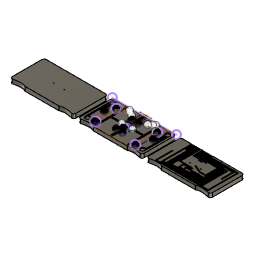
Arduino Foot Board V1.0 v3 (Autodesk Fusion 360 design; units mm, degrees)
Autodesk Fusion 360 part; units mm, degrees
(part 1 of 3)
sketch "TopZone" plane through (0, 0, 0) normal (0, 0, 1) x (1, 0, 0)
  line L0 (139.9424, 75.345) -> (-140.0576, 75.345)
  line L1 (-140.0576, 75.345) -> (-140.0576, -74.655)
  line L2 (-140.0576, -74.655) -> (139.9424, -74.655)
  line L3 (139.9424, -74.655) -> (139.9424, 75.345)
  line L4 (-0.0576, 75.345) -> (-0.0576, -74.655) construction
  line L5 (-140.0576, 0.345) -> (139.9424, 0.345) construction
  circle A0 centre (0, 0) radius 20
  circle A1 centre (0, 0) radius 27.5
  line L6 (-0.0576, 71.8935) -> (69.9424, 71.8935) construction
  line L7 (-0.0576, 71.8935) -> (-70.0576, 71.8935) construction
  line L8 (69.9424, 71.8935) -> (69.9424, -74.655)
  line L9 (69.9424, 71.8935) -> (69.9424, 75.345)
  line L10 (-70.0576, 71.8935) -> (-70.0576, 75.345)
  line L11 (-70.0576, 71.8935) -> (-70.0576, -74.655)
  line L12 (-8.6592, 0.345) -> (-8.6592, 2.845) construction
  line L13 (-8.6592, 0.345) -> (-8.6592, -2.155) construction
  line L14 (-27.3524, 2.845) -> (-70.0576, 2.845)
  line L15 (27.3524, 2.845) -> (69.9424, 2.845)
  line L16 (-27.4154, -2.155) -> (-70.0576, -2.155)
  line L17 (27.4154, -2.155) -> (69.9424, -2.155)
  line L18 (-0.0576, 7.4133) -> (2.4424, 7.4133) construction
  line L19 (-0.0576, 7.4133) -> (-5.0576, 7.4133) construction
  line L20 (4.9424, 27.0522) -> (4.9424, 75.345)
  line L21 (-5.0576, 27.0309) -> (-5.0576, 74.7158)
  line L22 (2.4424, -27.3913) -> (2.4424, -74.655)
  line L23 (-2.4424, -27.3913) -> (-2.4424, -74.655)
  line L24 (-0.0576, 48.2777) -> (4.9424, 48.2777) construction
  line L25 (-0.0576, 48.2777) -> (-5.0576, 48.2777) construction
  line L26 (41.5082, 0.345) -> (41.5082, 2.845) construction
  line L27 (41.5082, 0.345) -> (41.5082, -2.155) construction
  line L28 (-2.4424, -51.0232) -> (-0.0576, -51.0232) construction
  line L29 (-0.0576, -51.0232) -> (2.4424, -51.0232) construction
  line L30 (-47.1449, 0.345) -> (-47.1449, 2.845) construction
  line L31 (-47.1449, 0.345) -> (-47.1449, -2.155) construction
  line L32 (-0.0576, 41.5581) -> (85.9424, 41.5581) construction
  line L33 (-0.0576, 41.5581) -> (-86.0576, 41.5581) construction
  line L34 (-78.5277, 75.345) -> (-78.5277, 41.345) construction
  line L35 (-0.0576, -53.0508) -> (85.9424, -53.0508) construction
  line L36 (-86.0576, -53.0508) -> (-0.0576, -53.0508) construction
  line L37 (-80.4186, -74.655) -> (-80.4186, -54.655) construction
  line L38 (74.9056, 7.4117) -> (139.9424, 7.4117) construction
  line L39 (-75.019, 7.4166) -> (-140.0576, 7.4166) construction
  circle A2 centre (107.424, 7.4117) radius 12.5
  circle A3 centre (-107.5383, 7.4166) radius 12.5
  line L40 (-120.0383, 7.4166) -> (-120.0383, 57.4402) construction
  line L41 (-120.0383, 7.4166) -> (-120.0383, -52.5834) construction
  circle A4 centre (-120.0383, 57.4402) radius 10
  circle A5 centre (-120.0383, -52.5834) radius 10
  line L42 (-130.0383, -52.5834) -> (-130.0383, -52.5836)
  line L43 (-130.0383, 57.4402) -> (-130.0383, -52.5834)
  line L44 (-120.0383, 7.4166) -> (-120.0383, 47.4402)
  line L45 (-115.0383, 17.4167) -> (-115.0383, 47.4132)
  line L46 (-125.0305, 48.7754) -> (-125.0305, -43.9186)
  line L47 (-134.9926, -52.9708) -> (-134.9926, -52.2027)
  line L48 (-115.0383, 47.4132) -> (-115.0383, 48.7799)
  line L49 (119.924, 7.4117) -> (119.924, 57.4123) construction
  line L50 (119.924, 7.4117) -> (119.924, -52.5883) construction
  circle A6 centre (119.924, 57.4112) radius 10
  circle A7 centre (119.924, -52.5883) radius 10
  line L51 (129.924, -52.5895) -> (129.924, 57.4112)
  line L52 (119.924, 7.4117) -> (119.924, 47.4112)
  line L53 (114.9249, 17.411) -> (114.9249, 47.4133)
  line L54 (124.9251, -43.9287) -> (124.9251, 48.7516)
  line L55 (114.9249, 47.4133) -> (114.9249, 48.7504)
  line L56 (2.4424, -74.655) -> (13.049, -64.0484) construction
  line L57 (2.4424, -74.655) -> (17.5, -74.655) construction
  line L58 (-2.4424, -74.655) -> (-13.049, -64.0484) construction
  line L59 (-2.4424, -74.655) -> (12.5, -74.655) construction
  line L60 (4.9424, 75.345) -> (15.549, 64.7384) construction
  line L61 (4.9424, 75.345) -> (17.5, 75.345) construction
  line L62 (-5.0576, 74.7158) -> (-15.6642, 64.1092) construction
  line L63 (-5.0576, 74.7158) -> (12.5, 74.7158) construction
  circle A8 centre (13.049, -34.0489) radius 1.55
  circle A9 centre (-13.049, -34.0489) radius 1.55
  circle A10 centre (13.049, 34.7379) radius 1.55
  circle A11 centre (-13.1642, 34.387) radius 1.55
  circle A12 centre (-107.5383, 7.4166) radius 1.55
  circle A13 centre (107.424, 7.4117) radius 1.55
  circle A14 centre (0, 0) radius 1.55
  circle A15 centre (0, 0) radius 4
  circle A16 centre (13.049, -34.0489) radius 4
  circle A17 centre (-13.049, -34.0489) radius 4
  circle A18 centre (13.049, 34.7379) radius 4
  circle A19 centre (-13.1642, 34.387) radius 4
  circle A20 centre (107.424, 7.4117) radius 4
  circle A21 centre (-107.5383, 7.4166) radius 4
  line L64 (-75.019, 71.8935) -> (-75.019, -74.6555)
  line L65 (74.9056, 71.8935) -> (74.9056, -74.6555)
  line L66 (74.9056, 71.8935) -> (74.9056, 75.345)
  line L67 (-75.019, 71.8935) -> (-75.019, 75.345)
  line L68 (-5.0576, 74.7158) -> (-5.0576, 75.345)
  line L69 (74.9056, 7.4117) -> (-75.019, 7.4166) construction
  line L70 (-13.1642, 64.387) -> (-13.1642, 44.387) construction
  line L71 (13.049, 64.7379) -> (13.049, 44.7379) construction
  line L72 (-13.049, -64.0489) -> (-13.049, -44.0489) construction
  line L73 (13.049, -64.0489) -> (13.049, -44.0489) construction
  point P0 (-0.0576, -74.655)
  point P1 (-0.0576, 75.345)
  point P2 (139.9424, 0.345)
  point P3 (-140.0576, 0.345)
  dimension "d1" = 280
  dimension "d2" = 150
  dimension "d3" = 40
  dimension "d4" = 55
  dimension "d5" = 70
  dimension "d6" = 70
  dimension "d9" = 2.5
  dimension "d10" = 2.5
  dimension "d11" = 5
  dimension "d12" = 5
  dimension "d13" = 5
  dimension "d14" = 2.5
  dimension "d15" = 2.5
  dimension "d16" = 2.5
  dimension "d18" = 2.5
  dimension "d19" = 2.5
  dimension "d20" = 86
  dimension "d24" = 34
  dimension "d25" = 20
  dimension "d26" = 25
  dimension "d27" = 25
  dimension "d29" = 60
  dimension "d30" = 20
  dimension "d31" = 20
  dimension "d35" = 60
  dimension "d36" = 20
  dimension "d37" = 20
  dimension "d40" = 15
  dimension "d41" = 45
  dimension "d42" = 135
  dimension "d43" = 15
  dimension "d44" = 15
  dimension "d45" = 45
  dimension "d46" = 135
  dimension "d47" = 15
  dimension "d50" = 3.1
  dimension "d51" = 3.1
  dimension "d52" = 3.1
  dimension "d53" = 3.1
  dimension "d54" = 3.1
  dimension "d55" = 3.1
  dimension "d56" = 3.1
  dimension "d58" = 8
  dimension "d59" = 8
  dimension "d60" = 8
  dimension "d61" = 8
  dimension "d62" = 8
  dimension "d63" = 8
  dimension "d64" = 8
  dimension "d133" = 20
  dimension "d134" = 20
  dimension "d135" = 20
  dimension "d136" = 20
  constraint horizontal L0
  constraint perpendicular L0 L1
  constraint parallel L0 L2
  constraint parallel L1 L3
  constraint coincident A0.centre A1.centre
  constraint midpoint L0 P1
  constraint midpoint L2 P0
  constraint midpoint L1 P3
  constraint midpoint L3 P2
  constraint coincident L4 L6.start
  constraint perpendicular L4 L6
  constraint perpendicular L4 L7
  constraint coincident L2 L8.end
  constraint perpendicular L2 L8
  constraint coincident L0 L9.end
  constraint perpendicular L0 L9
  constraint coincident L0 L10.end
  constraint perpendicular L0 L10
  constraint coincident L2 L11.end
  constraint perpendicular L2 L11
  constraint coincident L5 L12.start
  constraint perpendicular L5 L12
  constraint perpendicular L5 L13
  constraint equal L12 L13
  constraint coincident A1 L14.start
  constraint coincident L11 L14.end
  constraint perpendicular L11 L14
  constraint coincident A1 L15.start
  constraint coincident L8 L15.end
  constraint perpendicular L8 L15
  constraint coincident A1 L16.start
  constraint coincident L11 L16.end
  constraint perpendicular L11 L16
  constraint coincident A1 L17.start
  constraint coincident L8 L17.end
  constraint perpendicular L8 L17
  constraint coincident L4 L18.start
  constraint perpendicular L4 L18
  constraint perpendicular L4 L19
  constraint coincident A1 L20.start
  constraint coincident L0 L20.end
  constraint perpendicular L0 L20
  constraint coincident A1 L21.start
  constraint perpendicular L19 L21
  constraint coincident A1 L22.start
  constraint coincident L2 L22.end
  constraint perpendicular L2 L22
  constraint coincident A1 L23.start
  constraint coincident L2 L23.end
  constraint perpendicular L2 L23
  constraint coincident L4 L24.start
  constraint coincident L20 L24.end
  constraint perpendicular L20 L24
  constraint coincident L21 L25.end
  constraint perpendicular L21 L25
  constraint coincident P0 L4.end
  constraint coincident P1 L4.start
  constraint coincident P2 L5.end
  constraint coincident P3 L5.start
  constraint coincident L5 L26.start
  constraint coincident L15 L26.end
  constraint perpendicular L15 L26
  constraint coincident L17 L27.end
  constraint perpendicular L17 L27
  constraint midpoint L23 L28.start
  constraint coincident L4 L28.end
  constraint perpendicular L23 L28
  constraint midpoint L22 L29.end
  constraint perpendicular L22 L29
  constraint coincident L5 L30.start
  constraint coincident L14 L30.end
  constraint perpendicular L14 L30
  constraint coincident L16 L31.end
  constraint perpendicular L16 L31
  constraint coincident L4 L32.start
  constraint perpendicular L32 L65
  constraint perpendicular L33 L64
  constraint coincident L0 L34.start
  constraint perpendicular L0 L34
  constraint coincident L4 L35.start
  constraint perpendicular L35 L65
  constraint perpendicular L4 L36
  constraint equal L32 L33
  constraint equal L32 L35
  constraint equal L32 L36
  constraint coincident L2 L37.start
  constraint perpendicular L36 L37
  constraint coincident L38.start L65
  constraint coincident L3 L38.end
  constraint perpendicular L3 L38
  constraint coincident L39.start L64
  constraint coincident L1 L39.end
  constraint perpendicular L1 L39
  constraint midpoint L38 A2.centre
  constraint midpoint L39 A3.centre
  constraint coincident A3 L40.start
  constraint coincident L39 L40.start
  constraint perpendicular L39 L40
  constraint perpendicular L5 L41
  constraint coincident L40.end A4.centre
  constraint coincident L41.end A5.centre
  constraint coincident A5 L42.start
  constraint coincident A5 L42.end
  constraint vertical L42
  constraint coincident A4 L43.start
  constraint perpendicular L5 L43
  constraint coincident A4 L44.end
  constraint coincident L40 L44.end
  constraint parallel L43 L46
  constraint parallel L42 L47
  constraint coincident A4 L46.start
  constraint coincident A5 L46.end
  constraint parallel L44 L45
  constraint coincident A3 L45.start
  constraint coincident A4 L48.end
  constraint parallel L45 L48
  constraint tangent A4 L43
  constraint tangent A5 L43
  constraint coincident A2 L49.start
  constraint coincident L38 L49.start
  constraint perpendicular L38 L49
  constraint perpendicular L38 L50
  constraint coincident L50.end A7.centre
  constraint coincident A7 L51.start
  constraint coincident A6 L51.end
  constraint tangent A6 L51
  constraint coincident A6 L52.end
  constraint perpendicular L38 L52
  constraint coincident A6 L55.end
  constraint parallel L53 L55
  constraint parallel L51 L54
  constraint coincident A6 L54.end
  constraint parallel L52 L53
  constraint coincident A2 L53.start
  constraint coincident A7 L54.start
  constraint horizontal L57
  constraint horizontal L59
  constraint horizontal L61
  constraint horizontal L63
  constraint concentric A3 A12
  constraint concentric A2 A13
  constraint concentric A1 A14
  constraint concentric A0 A15
  constraint concentric A8 A16
  constraint concentric A9 A17
  constraint concentric A10 A18
  constraint concentric A11 A19
  constraint concentric A13 A20
  constraint concentric A3 A21
  constraint parallel L8 L65
  constraint parallel L11 L64
  constraint coincident L0 L66.end
  constraint perpendicular L0 L66
  constraint coincident L0 L67.end
  constraint perpendicular L0 L67
  constraint coincident L0 L68.end
  constraint perpendicular L0 L68
  constraint vertical L70
  constraint vertical L71
  constraint perpendicular L36 L72
  constraint vertical L73
  measures "d1" distance of L1.end L2.end
  measures "d2" distance of L0.end L1.end
  measures "d3" diameter of A0
  measures "d4" diameter of A1
  measures "d5" distance of L6.start L6.end
  measures "d6" distance of L6.start L7.end
  measures "d9" distance of L12.start L12.end
  measures "d10" distance of L18.start L18.end
  measures "d11" distance of L18.start L19.end
  measures "d12" distance of L24.start L24.end
  measures "d13" distance of L24.start L25.end
  measures "d14" distance of L26.start L26.end
  measures "d15" distance of L26.start L27.end
  measures "d16" distance of L30.start L30.end
  measures "d18" distance of L30.start L31.end
  measures "d19" distance of L28.end L29.end
  measures "d20" distance of L32.start L32.end
  measures "d24" distance of L34.start L34.end
  measures "d25" distance of L37.start L37.end
  measures "d26" diameter of A2
  measures "d27" diameter of A3
  measures "d29" distance of L40.start L41.end
  measures "d30" diameter of A4
  measures "d31" diameter of A5
  measures "d35" distance of L49.start L50.end
  measures "d36" diameter of A6
  measures "d37" diameter of A7
  measures "d40" distance of L22.end L56.end
  measures "d41" angle of L56 L57
  measures "d42" angle of L58 L59
  measures "d43" distance of L23.end L58.end
  measures "d44" distance of L20.end L60.end
  measures "d45" angle of L60 L61
  measures "d46" angle of L62 L63
  measures "d47" distance of L21.end L62.end
  measures "d50" diameter of A8
  measures "d51" diameter of A9
  measures "d52" diameter of A10
  measures "d53" diameter of A11
  measures "d54" diameter of A12
  measures "d55" diameter of A13
  measures "d56" diameter of A14
  measures "d58" diameter of A15
  measures "d59" diameter of A16
  measures "d60" diameter of A17
  measures "d61" diameter of A18
  measures "d62" diameter of A19
  measures "d63" diameter of A20
  measures "d64" diameter of A21
  measures "d133" distance of L70.start L70.end
  measures "d134" distance of L71.start L71.end
  measures "d135" distance of L72.start L72.end
  measures "d136" distance of L73.start L73.end
sketch "LightResistorMeasurement" plane through (0, 0, 0) normal (0, 0, 1) x (1, 0, 0) in component "LightResistor v3"
  line L0 (0, 0) -> (0.0874, 0)
  line L1 (0, 0) -> (0, 2) construction
  line L2 (0, 0) -> (0, -2) construction
  line L3 (0, 2) -> (1.5, 2)
  line L4 (0, 2) -> (-1.5, 2)
  line L5 (0, -2) -> (1.5, -2)
  line L6 (0, -2) -> (-1.5, -2)
  arc A0 (-1.5, 2) -> (-1.5, -2) centre (0, 0) ccw
  arc A1 (1.5, -2) -> (1.5, 2) centre (0, 0) ccw
  line L7 (0, 0) -> (2, 0) construction
  line L8 (0, 0) -> (-2, 0) construction
  circle A2 centre (-1.7, 0) radius 0.3
  circle A3 centre (1.7, 0) radius 0.3
  dimension "d1_1" = 5
  dimension "d2_1" = 2
  dimension "d3_1" = 2
  dimension "d4_1" = 2
  dimension "d5_1" = 0.6
  dimension "d6_1" = 0.6
  constraint coincident L0.start L1.start
  constraint horizontal L0
  constraint perpendicular L0 L1
  constraint perpendicular L0 L2
  constraint equal L1 L2
  constraint perpendicular L1 L3
  constraint perpendicular L1 L4
  constraint coincident L5.end A0
  constraint perpendicular L2 L5
  constraint perpendicular L2 L6
  constraint concentric A0 A1
  constraint perpendicular L1 L7
  constraint perpendicular L2 L8
  constraint coincident L8.end A2
  constraint coincident L7.end A3
  measures "d1_1" diameter of A0
  measures "d2_1" distance of L0.start L1.end
  measures "d3_1" distance of L0.start L7.end
  measures "d4_1" distance of L0.start L8.end
  measures "d5_1" diameter of A2
  measures "d6_1" diameter of A3
extrude "Extrude1" add sketch "LightResistorMeasurement" along normal blind 1.8 contours L3 L4 L5 L6 A0 A1 | A2 | A3 makes body 1 in component "LightResistor v3"
extrude "Extrude2" add sketch "LightResistorMeasurement" against normal blind 24 contours A2 | A3 bodies 1 in component "LightResistor v3"
extrude "Extrude3" add sketch "LightResistorMeasurement" along normal blind 2 contours A2 | A3 bodies 1 in component "LightResistor v3"
sketch "WoodBoard" plane through (0, 0, 0) normal (0, 0, 1) x (1, 0, 0)
  line L0 (140, 75) -> (-140, 75)
  line L1 (-140, 75) -> (-140, -75)
  line L2 (-140, -75) -> (140, -75)
  line L3 (140, -75) -> (140, 75)
  line L4 (140, 75) -> (-140, -75) construction
  line L5 (-140, 75) -> (140, -75) construction
  dimension "d65" = 280
  dimension "d66" = 150
  constraint horizontal L0
  constraint perpendicular L0 L1
  constraint parallel L0 L2
  constraint parallel L1 L3
  constraint coincident L4 origin
  constraint coincident L5 origin
  measures "d65" distance of L1.end L2.end
  measures "d66" distance of L0.end L1.end
extrude "Extrude1'" add sketch "WoodBoard" against normal blind 18 separate body makes body 2
copy_body "CutPasteBodies1" bodies 1 removing the originals makes body 3
copy_body "CopyPasteBodies2" bodies 3 makes body 4
move_body "Move1" bodies 4 to x (1, 0, 0) y (0, 1, 0) z (0, 0, 1) at (-86.0576, 41.5581, 0)
copy_body "CopyPasteBodies3" bodies 3 makes body 5
move_body "Move2" bodies 5 to x (1, 0, 0) y (0, 1, 0) z (0, 0, 1) at (85.9424, 41.5581, 0)
copy_body "CopyPasteBodies4" bodies 3 makes body 6
move_body "Move3" bodies 6 to x (1, 0, 0) y (0, 1, 0) z (0, 0, 1) at (-86.0576, -53.0508, 0)
copy_body "CopyPasteBodies5" bodies 3 makes body 7
move_body "Move4" bodies 7 to x (1, 0, 0) y (0, 1, 0) z (0, 0, 1) at (85.9424, -53.0508, 0)
move_body "Move5" bodies 3 6 5 4 7 to x (1, 0, 0) y (0, 1, 0) z (0, 0, 1) at (0, 0, -1.8)
move_body "Move6" bodies 3 to x (1, 0, 0) y (0, 1, 0) z (0, 0, 1) at (0, -17, 0)
combine "Combine1" operation cut target body 2 tool bodies 3 4 5 6 7
sketch "LightResistorHoles" plane through (0, 0, 0) normal (0, 0, 1) x (1, 0, 0)
  circle A0 centre (-86.0576, 41.5581) radius 3
  circle A1 centre (85.9424, 41.5581) radius 3
  circle A2 centre (85.9424, -53.0508) radius 3
  circle A3 centre (-86.0576, -53.0508) radius 3
  circle A4 centre (-84.3576, 41.5581) radius 0.3
  circle A5 centre (-89.3076, 41.5581) radius 1.55
  circle A6 centre (-87.7576, 41.5581) radius 0.3
  circle A7 centre (-82.8076, -53.0508) radius 1.55
  circle A8 centre (-84.3576, -53.0508) radius 0.3
  circle A9 centre (-89.3065, -53.1098) radius 1.55
  circle A10 centre (-87.7576, -53.0508) radius 0.3
  circle A11 centre (89.1924, -53.0508) radius 1.55
  circle A12 centre (87.6424, -53.0508) radius 0.3
  circle A13 centre (82.6924, -53.0508) radius 1.55
  circle A14 centre (84.2424, -53.0508) radius 0.3
  circle A15 centre (89.1924, 41.5581) radius 1.55
  circle A16 centre (87.6424, 41.5581) radius 0.3
  circle A17 centre (82.6924, 41.5581) radius 1.55
  circle A18 centre (84.2424, 41.5581) radius 0.3
  circle A19 centre (2.6428, -15.7697) radius 1.55
  circle A20 centre (1.7, -17) radius 0.3
  circle A21 centre (-2.655, -15.7792) radius 1.55
  circle A22 centre (-1.7, -17) radius 0.3
  circle A23 centre (-82.8076, 41.5581) radius 1.55
  line L0 (-1.5, -15) -> (1.5, -15)
  line L1 (0, -15) -> (0, -13) construction
  circle A24 centre (0, 0) radius 20
  line L2 (0, -13) -> (15.1987, -13)
  line L3 (0, -13) -> (-15.1987, -13)
  line L4 (0, -13) -> (0, -11) construction
  line L5 (0, -11) -> (16.7033, -11)
  line L6 (0, -11) -> (-16.7033, -11)
  circle A25 centre (-86.0576, 41.5581) radius 4.8
  circle A26 centre (-86.0576, 41.5581) radius 6.5
  circle A27 centre (-86.0576, -53.0508) radius 4.8
  circle A28 centre (-86.0576, -53.0508) radius 6.5
  circle A29 centre (85.9424, -53.0508) radius 4.7714
  circle A30 centre (85.9424, -53.0508) radius 6.5
  circle A31 centre (85.9424, 41.5581) radius 4.8
  circle A32 centre (85.9424, 41.5581) radius 6.5
  point P0 (-86.0576, 41.5581)
  point P1 (85.9424, 41.5581)
  point P2 (85.9424, -53.0508)
  point P3 (-86.0576, -53.0508)
  dimension "d70" = 6
  dimension "d75" = 3.1
  dimension "d76" = 3.1
  dimension "d77" = 3.1
  dimension "d78" = 3.1
  dimension "d79" = 3.1
  dimension "d80" = 3.1
  dimension "d81" = 3.1
  dimension "d82" = 3.1
  dimension "d83" = 3.1
  dimension "d84" = 3.1
  dimension "d97" = 2
  dimension "d98" = 2
  dimension "d101" = 13
  constraint coincident P0 A0.centre
  constraint coincident P1 A1.centre
  constraint coincident P2 A2.centre
  constraint coincident P3 A3.centre
  constraint equal A0 A1
  constraint equal A0 A3
  constraint equal A0 A2
  constraint coincident A5 A6.centre
  constraint coincident A7 A8.centre
  constraint coincident A9 A10.centre
  constraint coincident A11 A12.centre
  constraint coincident A13 A14.centre
  constraint coincident A15 A16.centre
  constraint coincident A17 A18.centre
  constraint coincident A19 A20.centre
  constraint coincident A21 A22.centre
  constraint coincident A4.centre A23
  constraint midpoint L0 L1.start
  constraint perpendicular L0 L1
  constraint coincident A24 L2.end
  constraint perpendicular L1 L2
  constraint coincident A24 L3.end
  constraint perpendicular L1 L3
  constraint perpendicular L3 L4
  constraint coincident A24 L5.end
  constraint perpendicular L4 L5
  constraint coincident A24 L6.end
  constraint perpendicular L4 L6
  constraint tangent A23 A25
  constraint concentric A25 A26
  constraint concentric A3 A27
  constraint tangent A7 A27
  constraint concentric A2 A29
  constraint concentric A29 A30
  constraint concentric A1 A31
  constraint tangent A15 A31
  constraint concentric A1 A32
  constraint equal A26 A28
  constraint equal A26 A30
  constraint equal A26 A32
  measures "d70" diameter of A0
  measures "d75" diameter of A5
  measures "d76" diameter of A7
  measures "d77" diameter of A9
  measures "d78" diameter of A11
  measures "d79" diameter of A13
  measures "d80" diameter of A15
  measures "d81" diameter of A17
  measures "d82" diameter of A19
  measures "d83" diameter of A21
  measures "d84" diameter of A23
  measures "d97" distance of L1.start L1.end
  measures "d98" distance of L1.end L4.end
  measures "d101" diameter of A26
extrude "Extrude2'" cut sketch "LightResistorHoles" against normal blind 18 contours A0 A4 A23 | A0 A23 | A0 A5 A6 | A0 A5 | A4 A23 | A5 A6 | A1 A15 A16 | A1 A15 | A1 A17 A18 | A1 A17 | A15 A16 | A17 A18 | A2 A11 A12 | A2 A11 A29 | A2 A13 A14 | A2 A13 A29 | A11 A29 | A11 A12 | A13 A14 | A13 A29 | A3 A7 A8 | A3 A7 | A3 A9 A10 | A3 A9 | A7 A8 | A9 A10 | A19 A20 | A19 A20 | A21 A22 | A21 A22 picked at (-84.2555, 41.5581) picked at (-87.8544, 41.6205) picked at (87.7445, 41.5581) picked at (84.1456, 41.4957) picked at (87.7445, -53.0508) picked at (84.1456, -52.9883) picked at (-84.2555, -53.0508) picked at (-87.8583, -53.054) picked at (2.9931, -15.2653) picked at (1.7637, -16.9202) picked at (-3.0046, -15.274) picked at (-1.7629, -16.9195) bodies 2
extrude "Extrude3'" cut sketch "TopZone" against normal blind 1 contours L0 L2 L3 L65 L66 | L0 A1 L8 L9 L15 L20 | L2 A1 L8 L17 L22 | L0 A1 L10 L11 L14 L21 L68 | L2 A1 L11 L16 L23 | L0 L1 L2 L64 L67 | A0 bodies 2
extrude "Extrude4" cut sketch "TopZone" against normal blind 2 contours A15 | A16 | A17 | A18 | A19 | A20 | A21 bodies 2
extrude "Extrude5" cut sketch "TopZone" against normal blind 18 contours A8 | A9 | A10 | A11 | A12 | A13 | A14 bodies 2
extrude "Extrude6" cut sketch "TopZone" against normal blind 5 contours A2 | A2 A6 L52 L53 L55 | A6 | A6 A7 L51 L54 | A7 | A3 | A3 A4 L44 L45 L48 | A4 | A4 A5 L43 L46 | A5 bodies 2
extrude "Extrude7" cut sketch "TopZone" against normal blind 6 contours A20 | A21 bodies 2
extrude "Extrude8" add sketch "LightResistorHoles" against normal blind 3 contours A24 L2 L3 L5 L6 bodies 2
extrude "Extrude9" add sketch "LightResistorHoles" against normal blind 2 contours A26 | A28 | A30 | A32 bodies 2
sketch "RefPoints" plane through (0, 0, 0) normal (0, 0, 1) x (1, 0, 0)
  line L0 (-140, 75) -> (140, 75)
  line L1 (0, 0) -> (0, 81.0594) construction
  circle A0 centre (13.049, 34.7379) radius 1.55 construction
  line L2 (13.049, 34.7379) -> (13.049, 81.0594) construction
  circle A1 centre (-13.1642, 34.387) radius 1.55 construction
  line L3 (-13.1642, 34.387) -> (-13.1642, 81.0594) construction
  line L4 (0, 81.0594) -> (13.049, 81.0594) construction
  line L5 (0, 81.0594) -> (-13.1642, 81.0594) construction
  line L6 (6.5245, 81.0594) -> (6.5245, -71.9033) construction
  line L7 (6.5245, -71.9033) -> (78.613, -71.9033) construction
  line L8 (6.5245, -71.9033) -> (-78.7073, -71.9033) construction
  line L9 (82.8285, 41.5581) -> (82.8285, -53.0508) construction
  line L10 (82.8285, -53.0508) -> (82.8285, -71.9033) construction
  line L11 (78.613, -71.9033) -> (82.8285, -71.9033) construction
  arc A2 (-84.3286, -53.3494) -> (-84.3286, -52.7522) centre (-82.8076, -53.0508) ccw construction
  line L12 (-82.8598, 41.5581) -> (-82.8076, -53.0508) construction
  line L13 (-82.8076, -53.0508) -> (-82.7972, -71.9033) construction
  line L14 (-82.7972, -71.9033) -> (-78.7073, -71.9033) construction
  arc A3 (-88.2745, 42.7136) -> (-90.8576, 41.5581) centre (-89.3076, 41.5581) ccw construction
  line L15 (-89.3076, 41.5581) -> (-89.3076, 50.5559) construction
  arc A4 (90.7424, 41.5581) -> (88.1593, 42.7136) centre (89.1924, 41.5581) ccw construction
  line L16 (89.1924, 41.5581) -> (89.1924, 50.5559) construction
  arc A5 (88.1593, -54.2063) -> (90.7002, -53.4097) centre (89.1924, -53.0508) ccw construction
  line L17 (89.1924, -53.0508) -> (99.1924, -53.0508) construction
  arc A6 (-87.798, -52.7535) -> (-87.7753, -53.3502) centre (-89.3065, -53.1098) ccw construction
  line L18 (-89.3065, -53.1098) -> (-99.306, -53.2065) construction
  line L19 (-99.306, -53.2065) -> (-100.3741, 57.1678) construction
  circle A7 centre (-107.5383, 7.4166) radius 1.55 construction
  line L20 (-107.5383, 7.4166) -> (-107.5383, 65.4886) construction
  line L21 (99.1924, -53.0508) -> (99.1924, 59.674) construction
  circle A8 centre (107.424, 7.4117) radius 1.55 construction
  line L22 (107.424, 7.4117) -> (107.424, 65.1009) construction
  line L23 (107.424, 65.1009) -> (59.9835, 65.1009) construction
  line L24 (99.1924, 59.674) -> (50.873, 59.674) construction
  line L25 (89.1924, 50.5559) -> (38.3153, 50.5559) construction
  line L26 (-89.3076, 50.5559) -> (-31.1213, 50.5559) construction
  arc A9 (1.9547, -17.1586) -> (1.4807, -16.7953) centre (2.6428, -15.7697) ccw construction
  line L27 (2.6428, -15.7697) -> (6.5245, -15.7697) construction
  arc A10 (-1.4827, -16.7932) -> (-1.9531, -17.1611) centre (-2.655, -15.7792) ccw construction
  line L28 (-2.655, -15.7792) -> (-6.5367, -15.7792) construction
  line L29 (-6.5367, -15.7792) -> (-6.5367, 75.0019) construction
  line L30 (-6.5367, 75.0019) -> (-6.5821, 81.0594) construction
  line L31 (-100.3741, 57.1678) -> (-45.5643, 57.6981) construction
  line L32 (-107.5383, 65.4886) -> (-54.9128, 65.4886) construction
  circle A11 centre (-23.3525, 0) radius 1.55
  circle A12 centre (23.3525, 0) radius 1.55
  circle A13 centre (-13.049, -34.0489) radius 1.55
  line L33 (-13.049, -34.0489) -> (-23.049, -34.0489) construction
  circle A14 centre (13.049, -34.0489) radius 1.55
  line L34 (13.049, -34.0489) -> (23.049, -34.0489) construction
  line L35 (-23.049, -34.0489) -> (-23.049, 81.0594) construction
  line L36 (-23.049, 81.0594) -> (-13.1642, 81.0594) construction
  line L37 (23.049, -34.0489) -> (23.049, 81.0594) construction
  line L38 (23.049, 81.0594) -> (13.049, 81.0594) construction
  dimension "d107" = 10
  dimension "d108" = 10
  dimension "d109" = 3.1
  dimension "d110" = 3.1
  dimension "d131" = 10
  dimension "d132" = 10
  constraint coincident L1.start origin
  constraint perpendicular L0 L1
  constraint coincident A0.centre L2.start
  constraint perpendicular L0 L2
  constraint coincident A1.centre L3.start
  constraint perpendicular L0 L3
  constraint perpendicular L2 L4
  constraint perpendicular L3 L5
  constraint midpoint L4 L6.start
  constraint perpendicular L0 L6
  constraint perpendicular L6 L7
  constraint perpendicular L6 L8
  constraint perpendicular L8 L9
  constraint perpendicular L8 L10
  constraint perpendicular L10 L11
  constraint coincident A2.centre L12.end
  constraint parallel L8 L14
  constraint coincident A3.centre L15.start
  constraint perpendicular L8 L15
  constraint coincident A4.centre L16.start
  constraint coincident A5.centre L17.start
  constraint horizontal L17
  constraint coincident A6.centre L18.start
  constraint perpendicular L18 L19
  constraint vertical L20
  constraint coincident A7.centre L20.start
  constraint vertical L21
  constraint coincident A8.centre L22.start
  constraint perpendicular L17 L22
  constraint perpendicular L22 L23
  constraint perpendicular L21 L24
  constraint perpendicular L16 L25
  constraint perpendicular L15 L26
  constraint coincident A9.centre L27.start
  constraint coincident L6 L27.end
  constraint perpendicular L6 L27
  constraint coincident A10.centre L28.start
  constraint parallel L27 L28
  constraint equal L27 L28
  constraint vertical L29
  constraint midpoint L5 L30.end
  constraint perpendicular L19 L31
  constraint perpendicular L20 L32
  constraint coincident A13.centre L33.start
  constraint horizontal L33
  constraint coincident A14.centre L34.start
  constraint horizontal L34
  constraint perpendicular L5 L35
  constraint perpendicular L1 L36
  constraint perpendicular L0 L37
  constraint perpendicular L2 L38
  measures "d107" distance of A5.centre L17.end
  measures "d108" distance of A6.centre L18.end
  measures "d109" diameter of A11
  measures "d110" diameter of A12
  measures "d131" distance of A13.centre L33.end
  measures "d132" distance of A14.centre L34.end
extrude "Extrude10" cut sketch "RefPoints" against normal blind 2 contours A11 | A12 bodies 2
sketch "CutAround" plane through (0, 0, 0) normal (0, 0, 1) x (1, 0, 0)
  line L0 (-73.8561, -74.9863) -> (73.7471, -74.9863)
  line L1 (140, -64.9863) -> (140, 65)
  line L2 (130, 75) -> (-130, 75)
  line L3 (-140, 65) -> (-140, -64.9863)
  arc A0 (-130, 75) -> (-140, 65) centre (-130, 65) ccw
  arc A1 (140, 65) -> (130, 75) centre (130, 65) ccw
  arc A2 (-140, -64.9863) -> (-130.0009, -74.9863) centre (-130, -64.9863) ccw
  arc A3 (130.0008, -74.9863) -> (140, -64.9863) centre (130, -64.9863) ccw
  line L4 (-75.019, -74.655) -> (-140, -74.655)
  line L5 (-107.5095, -74.655) -> (-107.5095, -70.655) construction
  line L6 (139.9424, -74.655) -> (74.9056, -74.655)
  line L7 (107.424, -74.655) -> (107.424, -70.655) construction
  spline S0 degree 5 poles (-130.0009, -74.9863) (-129.11, -74.7683) (-127.3091, -74.3366) (-124.5504, -73.7016) (-120.7555, -72.8806) (-115.8051, -71.9105) (-110.6326, -71.0335) (-105.2246, -70.3193) (-99.5826, -69.885) (-93.7245, -69.8943) (-87.672, -70.5325) (-82.6907, -71.6937) (-78.8824, -72.9978) (-76.312, -74.069) (-75.019, -74.655) knots 0 0 0 0 0 0 0.1 0.2 0.3 0.4 0.5 0.6 0.7 0.8 0.9 1 1 1 1 1 1
  spline S1 degree 5 poles (130.0008, -74.9863) (129.1072, -74.7716) (127.3007, -74.3458) (124.5334, -73.7176) (120.7268, -72.9013) (115.7615, -71.9299) (110.5737, -71.0444) (105.1506, -70.3159) (99.4942, -69.8648) (93.6237, -69.8597) (87.5619, -70.492) (82.5765, -71.6598) (78.7676, -72.9773) (76.198, -74.0615) (74.9056, -74.655) knots 0 0 0 0 0 0 0.1 0.2 0.3 0.4 0.5 0.6 0.7 0.8 0.9 1 1 1 1 1 1
  line L8 (-75.019, -74.655) -> (-74.6817, -74.8079)
  line L9 (74.9056, -74.655) -> (74.5818, -74.8037)
  arc A4 (-74.6817, -74.8079) -> (-73.8561, -74.9863) centre (-73.8561, -72.9863) ccw
  arc A5 (73.7471, -74.9863) -> (74.5818, -74.8037) centre (73.7471, -72.9863) ccw
  line L10 (-74.6062, -73.7442) -> (-74.2689, -73.8971)
  arc A6 (-74.2689, -73.8971) -> (-73.8561, -73.9863) centre (-73.8561, -72.9863) ccw
  line L11 (-73.8561, -73.9863) -> (73.7471, -73.9863)
  arc A7 (73.7471, -73.9863) -> (74.1645, -73.895) centre (73.7471, -72.9863) ccw
  line L12 (74.4883, -73.7463) -> (74.1645, -73.895)
  spline S2 degree 3 poles (130.116, -73.9855) (125.372, -72.8483) (120.3191, -71.7486) (114.8797, -70.7875) (110.025, -69.9298) (104.8445, -69.1648) (99.3307, -68.9719) (93.8091, -68.7788) (87.9623, -69.2105) (81.9056, -70.9678) (79.4645, -71.676) (76.9901, -72.5973) (74.4883, -73.7463) knots 0.002638 0.002638 0.002638 0.002638 0.319613 0.319613 0.319613 0.602514 0.602514 0.602514 0.885821 0.885821 0.885821 1 1 1 1
  arc A8 (130.116, -73.9855) -> (139, -64.9863) centre (130, -64.9863) ccw
  line L13 (139, -64.9863) -> (139, 65)
  arc A9 (139, 65) -> (130, 74) centre (130, 65) ccw
  line L14 (130, 74) -> (-130, 74)
  arc A10 (-130, 74) -> (-139, 65) centre (-130, 65) ccw
  line L15 (-139, 65) -> (-139, -64.9863)
  arc A11 (-139, -64.9863) -> (-130.1182, -73.9855) centre (-130, -64.9863) ccw
  spline S3 degree 3 poles (-130.1182, -73.9855) (-125.3557, -72.8228) (-120.2812, -71.71) (-114.815, -70.7515) (-109.9113, -69.8915) (-104.6739, -69.1384) (-99.0955, -68.9821) (-93.5592, -68.8269) (-87.6968, -69.3115) (-81.6191, -71.1146) (-79.3104, -71.7996) (-76.9712, -72.6723) (-74.6062, -73.7442) knots 0.00269 0.00269 0.00269 0.00269 0.321768 0.321768 0.321768 0.608009 0.608009 0.608009 0.892088 0.892088 0.892088 1 1 1 1
  point P0 (-140, -75)
  point P1 (140, 75)
  dimension "d113" = 10
  dimension "d114" = 10
  dimension "d115" = 4
  dimension "d117" = 2
  dimension "d118" = 2
  dimension "d119" = -1
  constraint horizontal L0
  constraint vertical L1
  constraint horizontal L2
  constraint vertical L3
  constraint tangent L3 A0
  constraint tangent L2 A0
  constraint tangent L2 A1
  constraint tangent L1 A1
  constraint equal A0 A1
  constraint tangent L3 A2
  constraint tangent L0 A2
  constraint tangent L0 A3
  constraint tangent L1 A3
  constraint equal A2 A3
  constraint midpoint L4 L5.start
  constraint perpendicular L0 L5
  constraint midpoint L6 L7.start
  constraint perpendicular L0 L7
  constraint coincident L4.start S0.end
  constraint coincident L6.end S1.end
  constraint equal L5 L7
  constraint tangent L8 A4
  constraint tangent L0 A4
  constraint tangent L9 A5
  constraint tangent L0 A5
  measures "d113" radius of A0
  measures "d114" radius of A2
  measures "d115" distance of L5.start L5.end
  measures "d117" radius of A4
  measures "d118" radius of A5
extrude "Extrude11" cut sketch "CutAround" against normal blind 18 contours L10 A6 L11 A7 L12 S2 A8 L13 A9 L14 A10 L15 A11 S3 keep common part bodies 2
extrude "Extrude12" add sketch "RefPoints" along normal blind 1 separate body contours A11 | A12 makes body 8 at (24.9006, -0.0773, 0.6667) makes body 9 at (-21.8044, -0.0773, 0.6667)
move_body "Move10" bodies 8 9 to x (1, 0, 0) y (0, 1, 0) z (0, 0, 1) at (0, 0, -18)
combine "Combine2" operation cut target body 2 tool bodies 8 9